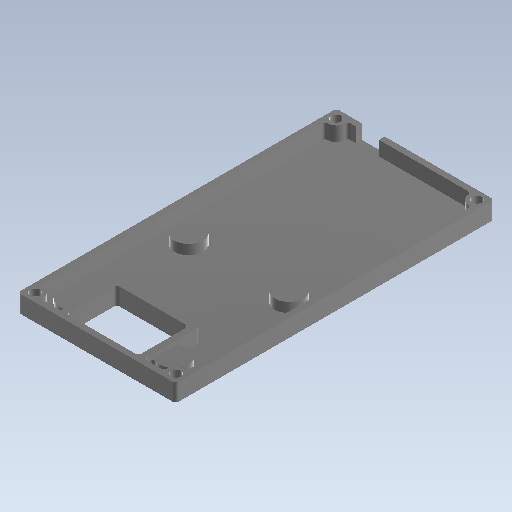
# Autodesk Inventor part: Circuit_protection_01
Saved by Autodesk Inventor 2020 (Build 240168000, 168)
## iProperties
Created: 2021-05-13
Part Number: Circuit_protection_01
Material: アセタール樹脂、黒
Document SubType Name: Modeling
Designer: Masato Kubotera
Density: 1.425 g/cm^3
Appearance: 滑らか - 黒
Mass: 13.7694 g
Surface Area: 157.492 cm^2
Volume: 9.66276 cm^3
Author: Masato Kubotera
Title: Circuit_protection_01
Autodesk Inventor part; units mm, degrees
ref_plane "YZ Plane" through (0, 0, 0) normal (1, 0, 0) x (0, 1, 0)
ref_plane "XZ Plane" through (0, 0, 0) normal (0, 1, 0) x (-1, 0, 0)
ref_plane "XY Plane" through (0, 0, 0) normal (0, 0, 1) x (1, 0, 0)
derived "Cockpit_horizontal_frame_02.ipt"
sketch "スケッチ1" plane through (0, 0, 0) normal (0, 0, 1) x (1, 0, 0)
  line L0 (-28, 65) -> (28, 65) construction
  line L1 (28, 65) -> (28, 47.1) construction
  line L2 (-28, -65) -> (-28, -47.1) construction
  line L3 (-28, 65) -> (28, -65) construction
  line L4 (28, 65) -> (-28, -65) construction
  line L5 (-28, 45) -> (-33, 45) construction
  line L6 (-33, 15) -> (-28, 15) construction
  line L7 (-33, 15) -> (-33, 45) construction
  line L8 (-28, -15) -> (-33, -15) construction
  line L9 (-33, -15) -> (-33, -45) construction
  line L10 (-33, -45) -> (-28, -45) construction
  arc A0 (-28, 45) -> (-28, 47.1) centre (-28, 46.05) ccw construction
  arc A1 (-28, 12.9) -> (-28, 15) centre (-28, 13.95) ccw construction
  arc A2 (-28, -15) -> (-28, -12.9) centre (-28, -13.95) ccw construction
  arc A3 (-28, -47.1) -> (-28, -45) centre (-28, -46.05) ccw construction
  line L11 (-28, 47.1) -> (-28, 65) construction
  line L12 (-28, 12.9) -> (-28, 15) construction
  line L13 (-28, -12.9) -> (-28, 12.9) construction
  line L14 (-28, -47.1) -> (-28, -45) construction
  line L15 (0, 65) -> (0, -65) construction
  arc A4 (28, -45) -> (28, -47.1) centre (28, -46.05) ccw construction
  line L16 (33, -45) -> (28, -45) construction
  line L17 (33, -15) -> (33, -45) construction
  line L18 (28, -15) -> (33, -15) construction
  arc A5 (28, -12.9) -> (28, -15) centre (28, -13.95) ccw construction
  arc A6 (28, 15) -> (28, 12.9) centre (28, 13.95) ccw construction
  line L19 (33, 15) -> (33, 45) construction
  line L20 (33, 15) -> (28, 15) construction
  line L21 (28, 45) -> (33, 45) construction
  arc A7 (28, 47.1) -> (28, 45) centre (28, 46.05) ccw construction
  line L22 (28, 47.1) -> (28, 45) construction
  line L23 (28, 12.9) -> (28, -12.9) construction
  line L24 (28, -47.1) -> (28, -65) construction
  line L25 (28, -12.9) -> (28, -15) construction
  line L26 (-28, -15) -> (-28, -12.9) construction
  line L27 (-28, -45) -> (-28, -15) construction
  line L28 (28, -15) -> (28, -45) construction
  line L29 (28, -45) -> (28, -47.1) construction
  line L30 (-20, -25) -> (-15, -25) construction
  line L31 (-15, -25) -> (-15, -45) construction
  line L32 (-15, -45) -> (-20, -45) construction
  line L33 (-20, -45) -> (-20, -25) construction
  line L34 (-20, -25) -> (-15, -45) construction
  line L35 (-15, -25) -> (-20, -45) construction
  line L36 (-20, 2.5) -> (-15, 2.5) construction
  line L37 (-15, 2.5) -> (-15, -72.5) construction
  line L38 (-15, -72.5) -> (-20, -72.5) construction
  line L39 (-20, -72.5) -> (-20, 2.5) construction
  line L40 (-20, 2.5) -> (-15, -72.5) construction
  line L41 (-15, 2.5) -> (-20, -72.5) construction
  circle A8 centre (-17.5, -55) radius 1.55 construction
  line L42 (-20, -35) -> (-15, -35) construction
  line L43 (-17.5, 2.5) -> (-17.5, -72.5) construction
  circle A9 centre (-17.5, -15) radius 1.55 construction
  circle A10 centre (17.5, -15) radius 1.55 construction
  circle A11 centre (17.5, -55) radius 1.55 construction
  line L44 (28, -65) -> (12.5, -65) construction
  line L45 (-12.5, -62.5) -> (-12.5, -45) construction
  line L46 (-12.5, -45) -> (0, -45) construction
  line L47 (12.5, -45) -> (0, -45) construction
  line L48 (12.5, -62.5) -> (12.5, -45) construction
  line L49 (-12.5, -65) -> (-28, -65) construction
  line L50 (12.5, -65) -> (-12.5, -65) construction
  line L51 (-28, 45) -> (-28, 47.1) construction
  line L52 (-28, 15) -> (-28, 45) construction
  line L53 (28, 15) -> (28, 12.9) construction
  line L54 (28, 45) -> (28, 15) construction
  circle A12 centre (-24.5, 43.5) radius 1.25 construction
  line L55 (-28, 0) -> (28, 0) construction
  line L56 (-28, 46.5) -> (28, 46.5) construction
  circle A13 centre (-24.5, -61.5) radius 1.25 construction
  circle A14 centre (24.5, 43.5) radius 1.25 construction
  circle A15 centre (24.5, -61.5) radius 1.25 construction
  circle A16 centre (-17.5, -55) radius 3 construction
  line L57 (-27.5, 46.5) -> (27.5, 46.5)
  line L58 (27.5, -64.5) -> (-27.5, -64.5)
  line L59 (-27.5, -64.5) -> (-27.5, 46.5)
  circle A17 centre (-24.5, -61.5) radius 1.75
  arc A18 (-21.6716, -62.5) -> (-25.5, -58.6716) centre (-24.5, -61.5) ccw
  circle A19 centre (24.5, -61.5) radius 1.75
  arc A20 (25.5, -58.6716) -> (21.6716, -62.5) centre (24.5, -61.5) ccw
  circle A21 centre (-17.5, -15) radius 3
  circle A22 centre (-17.5, -15) radius 5
  circle A23 centre (-17.5, -55) radius 3
  circle A24 centre (17.5, -15) radius 3
  circle A25 centre (17.5, -15) radius 5
  circle A26 centre (17.5, -55) radius 3
  line L60 (-12.5, -62.5) -> (-12.5, -45)
  line L61 (-12.5, -45) -> (12.5, -45)
  line L62 (21.6716, -62.5) -> (14.5, -62.5)
  line L63 (-14.5, -62.5) -> (-21.6716, -62.5)
  line L64 (12.5, -62.5) -> (12.5, -45)
  line L65 (-14.5, -43) -> (-14.5, -62.5)
  line L66 (-14.5, -43) -> (14.5, -43)
  line L67 (14.5, -43) -> (14.5, -62.5)
  line L68 (-25.5, -58.6716) -> (-25.5, 40.6716)
  line L69 (27.5, -64.5) -> (27.5, 46.5)
  line L70 (25.5, -58.6716) -> (25.5, 40.6716)
  line L71 (-27.5, -9) -> (27.5, -9) construction
  circle A27 centre (-24.5, 43.5) radius 1.75
  arc A28 (-25.5, 40.6716) -> (-21.6716, 44.5) centre (-24.5, 43.5) ccw
  circle A29 centre (24.5, 43.5) radius 1.75
  arc A30 (21.6716, 44.5) -> (25.5, 40.6716) centre (24.5, 43.5) ccw
  line L72 (-21.6716, 44.5) -> (21.6716, 44.5)
  circle A31 centre (-17.5, -55) radius 5
  circle A32 centre (17.5, -55) radius 5
  line L73 (-12.5, -62.5) -> (12.5, -62.5)
  line L74 (-18.605, 46.5) -> (-18.605, 44.5)
  line L75 (-14.605, 46.5) -> (-14.605, 44.5) construction
  line L76 (-10.605, 46.5) -> (-10.605, 44.5)
  line L77 (-12.5, -62.5) -> (12.5, -62.5)
  line L78 (-20, 41.5) -> (20, 41.5)
  line L79 (20, 2.5) -> (-20, 2.5)
  line L80 (-20, 2.5) -> (-20, 41.5)
  line L81 (20, 2.5) -> (20, 41.5)
  line L82 (-20.05, -43.5651) -> (-18.5651, -45.05) construction
  line L83 (-19.3075, -44.3075) -> (-20.05, -45.05) construction
  arc A33 (-20.05, -43.5651) -> (-18.5651, -45.05) centre (-19.3075, -44.3075) ccw
  line L84 (-20.05, -24.95) -> (-18.5651, -24.95) construction
  line L85 (-14.95, -24.95) -> (-14.95, -26.4349) construction
  line L86 (-14.95, -45.05) -> (-16.4349, -45.05) construction
  line L87 (-20.05, -45.05) -> (-20.05, -43.5651) construction
  line L88 (-20.05, -24.95) -> (-14.95, -45.05) construction
  line L89 (-14.95, -24.95) -> (-20.05, -45.05) construction
  arc A34 (-16.4349, -45.05) -> (-14.95, -43.5651) centre (-15.6925, -44.3075) ccw
  arc A35 (-14.95, -26.4349) -> (-16.4349, -24.95) centre (-15.6925, -25.6925) ccw
  arc A36 (-18.5651, -24.95) -> (-20.05, -26.4349) centre (-19.3075, -25.6925) ccw
  line L90 (-20.05, -43.5651) -> (-20.05, -26.4349)
  line L91 (-18.5651, -45.05) -> (-20.05, -45.05) construction
  line L92 (-16.4349, -45.05) -> (-18.5651, -45.05)
  line L93 (-14.95, -43.5651) -> (-14.95, -45.05) construction
  line L94 (-20.05, -26.4349) -> (-20.05, -24.95) construction
  line L95 (-18.5651, -24.95) -> (-16.4349, -24.95)
  line L96 (-16.4349, -24.95) -> (-14.95, -24.95) construction
  line L97 (-14.95, -26.4349) -> (-14.95, -43.5651)
  arc A37 (14.95, -43.5651) -> (16.4349, -45.05) centre (15.6925, -44.3075) ccw
  line L98 (16.4349, -45.05) -> (18.5651, -45.05)
  arc A38 (18.5651, -45.05) -> (20.05, -43.5651) centre (19.3075, -44.3075) ccw
  line L99 (20.05, -43.5651) -> (20.05, -26.4349)
  line L100 (14.95, -26.4349) -> (14.95, -43.5651)
  arc A39 (20.05, -26.4349) -> (18.5651, -24.95) centre (19.3075, -25.6925) ccw
  line L101 (18.5651, -24.95) -> (16.4349, -24.95)
  arc A40 (16.4349, -24.95) -> (14.95, -26.4349) centre (15.6925, -25.6925) ccw
  line L102 (-28, -65) -> (-28, -70)
  line L103 (-28, -70) -> (28, -70)
  line L104 (28, -70) -> (28, -65)
  point P0 (0, 0)
  point P1 (0, 0)
  point P2 (0, 0)
  point P3 (-17.5, -35)
  point P4 (20.3453, -61)
  point P5 (25.5, 40.6716)
  point P6 (-12.5, -64.5)
  point P7 (-12.5, -55)
  point P8 (-14.5, -59)
  point P9 (14.5, -59)
  point P10 (12.5, -55)
  point P11 (12.5, -64.5)
  point P12 (-14.5, -51)
  point P13 (14.5, -51)
  point P14 (28, 45)
  point P15 (28, 45)
  dimension "d14" = 0.5
  dimension "d15" = 0.5
  dimension "d27" = 3.5
  dimension "d32" = 6
  dimension "d33" = 6
  dimension "d34" = 10
  dimension "d35" = 0
  dimension "d36" = 0
  dimension "d39" = 2
  dimension "d40" = 2
  dimension "d49" = 2
  dimension "d50" = 2
  dimension "d52" = 0.5
  dimension "d55" = 14.605
  dimension "d56" = 8
  measures "d15" distance between parallel lines of L49 L58
  measures "d27" diameter of A17
  measures "d32" diameter of A18
  measures "d33" diameter of A21
  measures "d34" diameter of A22
  measures "d35" distance between parallel lines of L45 L60
  measures "d36" distance between parallel lines of L61 L46
  measures "d39" distance between parallel lines of L65 L60
  measures "d40" distance between parallel lines of L61 L66
  measures "d49" distance between parallel lines of L59 L68
  measures "d50" distance between parallel lines of L58 L63
  measures "d52" distance between parallel lines of L24 L69
  measures "d55" distance between parallel lines of L15 L75
  measures "d56" distance between parallel lines of L74 L76
extrude "押し出し1" add sketch "スケッチ1" along normal blind 6 contours L57 L74 L72 A28 L68 A18 L63 L65 A31 L60 L73 L64 A32 L67 L62 A20 L70 A30 L76 L69 L58 L59 | L65 A31 | A32 L67 | L65 L66 L67 A32 L64 L61 L60 A31 picked at (-14.2204, -52.5988) picked at (14.2204, -57.4012)
extrude "押し出し2" add sketch "スケッチ1" along normal blind 1 contours L57 L76 L72 L74 | L72 A30 L70 A20 L62 L67 A32 L66 L65 A31 L63 A18 L68 A28 | L78 L81 L79 L80 | L90 A36 L95 A35 L97 A34 L92 A33 | L100 A40 L101 A39 L99 A38 L98 A37
extrude "押し出し3" add sketch "スケッチ1" along normal blind 4.4 contours A23 | A31 L65 | L65 A31 | A32 L67 | A26 | L67 A32 | A21 | A22 | A24 | A25
extrude "押し出し4" cut sketch "スケッチ1" along normal blind 3.5 contours A23 | A26 | A21 | A24
fillet "フィレット1" radius 1 24 edges at (21.6716, -62.5, 3.5) (14.5, -43, 3.5) (-21.6716, -62.5, 3.5) (-25.5, -58.6716, 3.5) (-14.5, -43, 3.5) (14.5, -62.5, 3.5) (-14.5, -62.5, 3.5) (-27.5, -64.5, 3) (-12.5, -45, 3) (12.5, -45, 3) (12.5, -62.5, 3) (27.5, -64.5, 3) (25.5, -58.6716, 3.5) (14.5, -59, 2.7) (14.5, -51, 2.7) (-14.5, -59, 2.7) (-14.5, -51, 2.7) (-27.5, 46.5, 3) (-25.5, 40.6716, 3.5) (-21.6716, 44.5, 3.5) (25.5, 40.6716, 3.5) (21.6716, 44.5, 3.5) (27.5, 46.5, 3) (-12.5, -62.5, 3)
equation "\"d15\" = d14"
equation "\"d39\" = d50"
equation "\"d40\" = d50"
equation "\"d50\" = d49"
equation "\"d19\" = d18"
equation "\"d18\" = 2"
